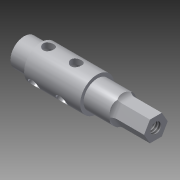
# Autodesk Inventor part: Ball Shisting Shaft Outline Sketch
Saved by Autodesk Inventor 2013 (Build 170138000, 138)
## iProperties
Created: 2013-06-04
Part Number: Ball Shisting Shaft Outline Sketch
Material: Aluminum 6061
Document SubType Name: Modeling
Designer: mvarma
Density: 1 g/cm^3
Author: mvarma
Autodesk Inventor part; units mm, degrees
ref_plane "YZ Plane" through (0, 0, 0) normal (1, 0, 0) x (0, 1, 0)
ref_plane "XZ Plane" through (0, 0, 0) normal (0, 1, 0) x (-1, 0, 0)
ref_plane "XY Plane" through (0, 0, 0) normal (0, 0, 1) x (1, 0, 0)
sketch "Sketch1" plane through (0, 0, 0) normal (0, 0, 1) x (1, 0, 0)
  line L0 (0, 0) -> (0, 5.5563) construction
  line L1 (0, 0) -> (7.9375, 0)
  line L2 (7.9375, 0) -> (8.1915, 0)
  line L3 (0, 6.35) -> (7.9375, 6.35)
  line L4 (7.9375, 6.35) -> (7.9375, 0) construction
  line L5 (0, 5.5563) -> (7.9375, 5.5563)
  line L6 (7.9375, 6.35) -> (7.9375, 7.9375)
  line L7 (7.9375, 7.9375) -> (33.9725, 7.9375)
  line L8 (33.9725, 0) -> (33.9725, 7.8403) construction
  line L9 (33.9725, 7.8403) -> (33.9725, 7.8403)
  line L10 (33.9725, 7.8403) -> (33.9725, 6.35)
  line L11 (33.9725, 0) -> (33.9725, 0)
  line L12 (33.9725, 6.35) -> (42.164, 6.35)
  line L13 (42.164, 6.35) -> (42.164, 0)
  line L14 (33.9725, 0) -> (34.2265, 0)
  line L15 (34.2265, 0) -> (39.6415, 0)
  line L16 (34.2265, 0) -> (34.2265, 6.35) construction
  line L17 (7.9375, 5.5563) -> (26.7144, 5.5563)
  line L18 (16.4059, 7.874) -> (17.6759, 7.874) construction
  line L19 (0, 3.1115) -> (42.164, 3.1115) construction
  line L20 (0, 5.1753) -> (42.164, 5.1753) construction
  line L21 (8.1915, 0) -> (8.1915, 7.9375) construction
  line L22 (8.1915, 0) -> (8.9852, 0)
  line L23 (8.9852, 0) -> (8.9852, 7.9375) construction
  line L24 (8.9852, 7.9375) -> (8.9852, 25.0214) construction
  line L25 (8.9852, 25.0214) -> (13.7477, 25.0214) construction
  line L26 (13.7477, 25.0214) -> (13.7477, 0) construction
  line L27 (13.7477, 0) -> (8.9852, 0)
  line L28 (13.7477, 17.4625) -> (21.082, 17.4625) construction
  line L29 (13.7477, 25.0214) -> (18.5102, 25.0214) construction
  line L30 (18.5102, 25.0214) -> (18.5103, 0) construction
  line L31 (18.5103, 0) -> (13.7477, 0)
  line L32 (21.082, 17.4625) -> (21.082, 0) construction
  line L33 (21.082, 0) -> (18.5103, 0)
  line L34 (21.082, 0) -> (21.8757, 0)
  line L35 (21.8757, 0) -> (21.8757, 14.2875) construction
  line L36 (21.8757, 14.2875) -> (21.082, 14.2875) construction
  line L37 (8.1915, 7.9375) -> (8.1915, 14.2875) construction
  line L38 (8.1915, 14.2875) -> (8.9852, 14.2875) construction
  line L39 (21.8757, 30.0415) -> (26.6382, 30.0415) construction
  line L40 (26.6382, 30.0415) -> (26.6382, 0) construction
  line L41 (26.6382, 0) -> (21.8757, 0)
  line L42 (26.6382, 30.0415) -> (31.4007, 30.0415) construction
  line L43 (31.4007, 30.0415) -> (31.4007, 0) construction
  line L44 (26.6382, 0) -> (31.4007, 0)
  line L45 (26.6382, 17.4625) -> (33.9725, 17.4625) construction
  line L46 (33.9725, 17.4625) -> (33.9725, 0) construction
  line L47 (33.9725, 0) -> (31.4007, 0)
  line L48 (21.8757, 14.2875) -> (21.8757, 30.0415) construction
  line L49 (33.9725, 0) -> (33.9725, 0)
  line L50 (11.3665, 25.0214) -> (11.3665, 0) construction
  line L51 (24.257, 30.0415) -> (24.257, 0) construction
  circle A0 centre (11.3665, 7.5565) radius 2.3813 construction
  circle A1 centre (11.3665, 5.4927) radius 2.3813 construction
  line L52 (8.9893, 7.874) -> (10.2593, 7.874) construction
  circle A2 centre (24.257, 5.4927) radius 2.3812 construction
  circle A3 centre (24.257, 7.5565) radius 2.3812 construction
  line L53 (23.0177, 7.874) -> (24.0459, 7.874) construction
  line L54 (14.6367, 5.1752) -> (12.573, 3.1115) construction
  line L55 (20.9867, 5.1752) -> (23.0505, 3.1115) construction
  line L56 (10.7315, 5.1752) -> (8.6677, 3.1115) construction
  line L57 (10.4775, 5.1752) -> (8.4137, 3.1115) construction
  line L58 (0, 3.5719) -> (8.8741, 3.5719) construction
  line L59 (0, 3.5719) -> (-1.5875, 3.5719) construction
  line L60 (-1.5875, 3.5719) -> (-1.5875, 6.35) construction
  line L61 (-1.5875, 6.35) -> (0, 6.35) construction
  line L62 (26.7144, 7.9375) -> (26.7144, 0) construction
  line L63 (24.892, 5.1752) -> (26.9557, 3.1115) construction
  line L64 (26.7144, 5.5563) -> (28.026, 3.3734)
  line L65 (16.8275, 5.1752) -> (18.8912, 3.1115) construction
  line L66 (37.5179, 3.1115) -> (37.5179, 0) construction
  line L67 (16.4782, 3.1115) -> (18.542, 5.1752) construction
  line L68 (69.3538, 20.0694) -> (73.1082, 25.272) construction
  line L69 (73.1082, 25.272) -> (79.491, 24.6219) construction
  line L70 (79.491, 24.6219) -> (82.1194, 18.7692) construction
  line L71 (82.1194, 18.7692) -> (78.365, 13.5666) construction
  line L72 (78.365, 13.5666) -> (71.9822, 14.2167) construction
  line L73 (71.9822, 14.2167) -> (69.3538, 20.0694) construction
  circle A4 centre (75.7366, 19.4193) radius 6.4158 construction
  line L74 (42.164, 5.5562) -> (53.7803, 5.5563) construction
  line L75 (53.7803, 5.5563) -> (53.7803, 0) construction
  line L76 (53.7803, 0) -> (42.164, 0) construction
  line L77 (28.026, 3.3734) -> (37.6145, 3.3734)
  line L78 (31.323, 0) -> (29.4534, 3.1115) construction
  line L79 (37.5179, 3.1115) -> (39.3875, 0) construction
  line L80 (37.7719, 3.1115) -> (39.6415, 0)
  line L81 (8.909, 7.9375) -> (8.909, 0) construction
  line L82 (37.7719, 3.1115) -> (37.6145, 3.3734)
  line L83 (0, 5.5563) -> (0, 6.35)
  line L84 (33.9725, 7.8403) -> (33.9725, 7.9375)
  line L85 (33.9725, 6.35) -> (33.9725, 0) construction
  line L86 (26.7144, 5.5563) -> (42.164, 5.5563) construction
  line L87 (28.026, 3.3734) -> (28.1834, 3.1115) construction
  line L88 (37.6145, 3.3734) -> (42.164, 3.3734) construction
  line L89 (39.6415, 0) -> (42.164, 0)
  point P0 (11.3665, 3.1115)
  point P1 (11.3665, 5.1753)
  point P2 (24.257, 5.1752)
  dimension "d78" = 4.7625
  dimension "d82" = 4.7625
  dimension "d116" = 12.8316
  dimension "d40" = 0.254
  dimension "d41" = 7.9375
  dimension "d42" = 6.35
  dimension "d43" = 5.5563
  dimension "d44" = 7.9375
  dimension "d46" = 7.8403
  dimension "d47" = 0
  dimension "d48" = 0.254
  dimension "d49" = 6.35
  dimension "d50" = 7.9375
  dimension "d53" = 1.27
  dimension "d54" = 0.0635
  dimension "d58" = 3.1115
  dimension "d61" = 5.1753
  dimension "d63" = 0.7937
  dimension "d64" = 4.7625
  dimension "d65" = 7.3342
  dimension "d66" = 17.4625
  dimension "d67" = 4.7625
  dimension "d68" = 0.7937
  dimension "d69" = 14.2875
  dimension "d70" = 14.2875
  dimension "d71" = 4.7625
  dimension "d72" = 4.7625
  dimension "d73" = 7.3342
  dimension "d74" = 17.4625
  dimension "d75" = 0
  dimension "d76" = 12.8905
  dimension "d77" = 0.381
  dimension "d80" = 0.0635
  dimension "d81" = 4.7625
  dimension "d83" = 0.381
  dimension "d84" = 0.0635
  dimension "d85" = 45
  dimension "d86" = 45
  dimension "d88" = 1.2065
  dimension "d89" = 6.35
  dimension "d90" = 3.2702
  dimension "d91" = 0.635
  dimension "d92" = 45
  dimension "d93" = 0.254
  dimension "d94" = 3.5719
  dimension "d95" = 0.4604
  dimension "d96" = 1.5875
  dimension "d97" = 2.7781
  dimension "d98" = 1.6034
  dimension "d99" = 3.9053
  dimension "d101" = 3.2702
  dimension "d102" = 4.9149
  dimension "d103" = 0.635
  dimension "d105" = 59
  dimension "d106" = 2.4977
  dimension "d107" = 6.35
  dimension "d108" = 45
  dimension "d109" = 8.0645
  dimension "d110" = 10.5622
  dimension "d114" = 6.35
  dimension "d115" = 11.1125
  dimension "d117" = 5.5563
  dimension "d118" = 3.1115
  dimension "d120" = 3.3734
  dimension "d121" = 59
  dimension "d122" = 1.27
  dimension "d123" = 59
  constraints: 176 end point, 45 perpendicular, 33 point on line, 16 parallel, 8 collinear, 6 horizontal, 5 vertical, 4 midpoint, 3 vertical alignment, 1 centre point, 1 coincident, 1 tangent, 46 other
  measures "d40" distance of L1.end L2.end
  measures "d41" distance of L0.start L1.end
  measures "d42" distance between parallel lines of L1 L3
  measures "d43" distance between parallel lines of L1 L5
  measures "d44" distance from line of L0.start L7
  measures "d46" distance from line of L8.start L9
  measures "d47" distance of L8.end L9.end
  measures "d48" distance of L11.start L14.end
  measures "d49" distance between parallel lines of L15 L12
  measures "d50" distance of L14.end L13.end
  measures "d53" distance of L18.start L18.end
  measures "d54" distance between parallel lines of L7 L18
  measures "d63" distance of L2.end L22.end
  measures "d64" distance of L24.end L25.end
  measures "d65" distance of L28.start L28.end
  measures "d66" distance between parallel lines of L27 L28
  measures "d67" distance of L25.end L29.end
  measures "d68" distance of L32.end L34.end
  measures "d69" distance between parallel lines of L34 L36
  measures "d70" distance between parallel lines of L22 L38
  measures "d71" distance of L39.start L39.end
  measures "d72" distance of L39.end L42.end
  measures "d73" distance of L45.start L45.end
  measures "d74" distance between parallel lines of L44 L45
  measures "d75" distance of L46.end L8.start
  measures "d76" distance between parallel lines of L51 L50
  measures "d77" distance from line of L7 point (11.366, 7.556)
  measures "d80" distance between parallel lines of L7 L52
  measures "d81" diameter of A2
  measures "d83" distance from line of L7 point (24.257, 7.556)
  measures "d84" distance between parallel lines of L7 L53
  measures "d85" angle to the sketch x axis of L54
  measures "d86" angle to the sketch x axis of L55
  measures "d88" distance of point (11.366, 3.111) L54.end
  measures "d89" distance of L55.start L54.start
  measures "d90" distance of L54.start point (11.366, 5.175)
  measures "d91" distance of point (11.366, 5.175) L56.start
  measures "d92" angle to the sketch x axis of L56
  measures "d93" distance of L56.start L57.start
  measures "d94" distance between parallel lines of L1 L58
  measures "d96" distance between parallel lines of L0 L60
  measures "d97" distance between parallel lines of L3 L58
  measures "d99" distance of L54.start L56.start
  measures "d101" distance of point (24.257, 5.175) L55.start
  measures "d102" diameter of L62 L51
  measures "d103" distance of point (24.257, 5.175) L63.start
  measures "d105" angle to the sketch x axis of L64
  measures "d106" distance of L78.end L63.end
  measures "d107" distance of L65.start L57.start
  measures "d108" angle to the sketch x axis of L65
  measures "d109" distance of L63.start L65.start
  measures "d110" distance of L66.start L63.end
  measures "d114" distance of L63.start L67.end
  measures "d115" distance between parallel lines of L72 L69
  measures "d117" distance between parallel lines of L76 L74
  measures "d120" distance between parallel lines of L47 L77
  measures "d121" angle of L44 L78
  measures "d122" distance of L87.end L78.end
  measures "d123" angle of L15 L79
revolve "Revolution1" add sketch "Sketch1" angle 360 about axis through (33.9725, 0, 0) along (-1, 0, 0)
sketch "Sketch3" plane through (0, 0, 0) normal (0, 1, 0) x (-1, 0, 0)
  circle A0 centre (-11.3665, 0) radius 2.4575
  line L0 (0, 0) -> (-11.3665, 0) construction
  circle A1 centre (-24.257, 0) radius 2.4574
  line L1 (-11.3665, 0) -> (-24.257, 0) construction
  dimension "d135" = 4.9149
  dimension "d137" = 11.3665
  dimension "d138" = 12.8905
  constraints: 4 end point, 2 centre point, 2 horizontal, 1 coincident, 1 equal radius
  measures "d135" diameter of A0
  measures "d137" distance of L0.start L0.end
  measures "d138" distance of L0.end A1.centre
extrude "Extrusion3" cut sketch "Sketch3" along normal blind 25.4
pattern_circular "Circular Pattern1" count 3 over 360 about axis through (-10, 0, 0) along (1, 0, 0) of "Extrusion3"
sketch "Sketch4" plane through (42.164, 0, 0) normal (1, 0, 0) x (0, 0, -1)
  circle A0 centre (0, 0) radius 6.35 projected
extrude "Extrusion4" add sketch "Sketch4" along normal blind 3.6068
sketch "Sketch9" plane through (45.7708, 0, 0) normal (1, 0, 0) x (0, 0, -1)
  circle A0 centre (0, 0) radius 6.35 projected
  line L0 (5.4993, 0) -> (2.7496, -4.7625)
  line L1 (2.7496, -4.7625) -> (-2.7496, -4.7625)
  line L2 (-2.7496, -4.7625) -> (-5.4993, 0)
  line L3 (-5.4993, 0) -> (-2.7496, 4.7625)
  line L4 (-2.7496, 4.7625) -> (2.7496, 4.7625)
  line L5 (2.7496, 4.7625) -> (5.4993, 0)
  dimension "d167" = 9.525
  constraints: 12 end point, 1 coincident, 1 horizontal, 13 other
  measures "d167" distance between parallel lines of L1 L4
extrude "Extrusion8" add sketch "Sketch9" along normal blind 15.4432 contours L0 L1 L2 L3 L4 L5
ref_plane "Work Plane4" through (45.7708, 0, 0) normal (1, 0, 0) x (0, 0, -1)
sketch "Sketch10" plane through (0, 0, 0) normal (0, 0, 1) x (1, 0, 0)
  line L0 (45.7708, 4.7625) -> (61.214, 4.7625) projected
  line L1 (45.7708, -6.35) -> (45.7708, 6.35) projected
  circle A0 centre (48.5204, 7.9375) radius 3.175
  line L2 (45.7708, 6.35) -> (45.7708, 4.7625)
  line L3 (48.5204, 4.7625) -> (45.7708, 4.7625)
  point P0 (0, 0)
  dimension "d170" = 6.35
  constraints: 4 end point, 2 collinear, 2 point on circle, 2 tangent, 1 centre point, 1 point on line
  measures "d170" diameter of A0
ref_plane "Work Plane3" through (45.7708, 4.7625, 2.7496) normal (0, 0.5, -0.8660254) x (1, 0, 0)
extrude "Extrusion9" add sketch "Sketch10" against normal up to surface contours L1 A0 L0 surface through (45.7708, 4.7625, 2.7496) normal (0, 0.5, -0.8660254)
mirror "Mirror2" about plane through (46.7746, 5.1475, 0) normal (0, 0, -1) of "Extrusion9"
pattern_circular "Circular Pattern3" count 6 over 360 about axis through (38.0682, 0, 0) along (1, 0, 0) of "Extrusion9", "Mirror2"
sketch "Sketch11" plane through (33.9725, 0, 0) normal (1, 0, 0) x (0, 0, -1)
  circle A0 centre (0, 0) radius 7.9375 projected
  circle A1 centre (0, 0) radius 6.35 projected
extrude "Extrusion10" cut sketch "Sketch11" along normal up to surface (27.2415 mm away)
sketch "Sketch12" plane through (61.214, 0, 0) normal (1, 0, 0) x (0, 0, -1)
  point P0 (0, 0)
  point P1 (0, 0)
  constraints: 1 coincident
hole "Hole2" at (61.214, 0, 0) direction (-1, 0, 0) diameter 4.9784 depth 14.2875 tip angle 118 thread size "1/4-20 UNC" class "2B" standard "ANSI Unified Screw Threads"
body "Solid1"
